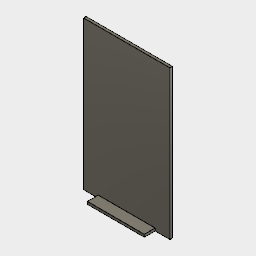
Separator (Autodesk Fusion 360 design; units mm, degrees)
Autodesk Fusion 360 part; units mm, degrees
sketch "Sketch1" plane through (0, 0, 0) normal (0, 1, 0) x (1, 0, 0)
  line L0 (0, 0) -> (31.94, 0)
  line L1 (31.94, 0) -> (31.94, 0.99)
  line L2 (31.94, 0.99) -> (0, 0.99)
  line L3 (0, 0.99) -> (0, 0)
extrude "Extrude1" add sketch "Sketch1" along normal blind 55
sketch "Sketch3" plane through (0, 0, 0) normal (0, -1, 0) x (1, 0, 0)
  line L0 (0, 0) -> (0, -0.99)
  line L1 (0, -0.99) -> (31.94, -0.99)
  line L2 (31.94, -0.99) -> (31.94, 0)
  line L3 (31.94, 0) -> (0, 0)
  line L4 (5.44, 0) -> (26.5, 0)
  line L5 (26.5, 0) -> (26.5, 4)
  line L6 (26.5, 4) -> (5.44, 4)
  line L7 (5.44, 4) -> (5.44, 0)
extrude "Extrude2" add sketch "Sketch3" against normal blind 1 contours L3 L4 L5 L6 L7
sketch "Sketch4" plane through (0, 0, 0) normal (0, 1, 0) x (1, 0, 0)
  line L0 (5.44, 0.99) -> (26.5, 0.99)
  line L1 (26.5, 0.99) -> (26.5, 4.99)
  line L2 (26.5, 4.99) -> (5.44, 4.99)
  line L3 (5.44, 4.99) -> (5.44, 0.99)
  line L4 (31.94, 0.99) -> (0, 0.99)
extrude "Extrude3" add sketch "Sketch4" along normal blind 1
